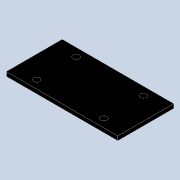
# Autodesk Inventor part: X Axis Belt Tentoner NON ADJUSTABLE Top
Saved by Autodesk Inventor 2022 (Build 260153000, 153)
## iProperties
Created: 2021-10-23
Part Number: X Axis Belt Tentoner NON ADJUSTABLE Top
Material: Generic
Document SubType Name: Modeling
Designer: Coy
Density: 1 g/cm^3
Appearance: Anodized - Black
Author: Coy
Autodesk Inventor part; units mm, degrees
ref_plane "YZ Plane" through (0, 0, 0) normal (1, 0, 0) x (0, 1, 0)
ref_plane "XZ Plane" through (0, 0, 0) normal (0, 1, 0) x (-1, 0, 0)
ref_plane "XY Plane" through (0, 0, 0) normal (0, 0, 1) x (1, 0, 0)
sketch "Sketch1" plane through (0, 0, 0) normal (0, 1, 0) x (-1, 0, 0)
  line L0 (0, 0) -> (93, 0)
  line L1 (93, 0) -> (93, 46.65)
  line L2 (93, 46.65) -> (0, 46.65)
  line L3 (0, 46.65) -> (0, 0)
  line L4 (74.5, 39.825) -> (18.5, 39.825) construction
  line L5 (18.5, 39.825) -> (18.5, 6.825) construction
  line L6 (18.5, 6.825) -> (74.5, 6.825) construction
  line L7 (74.5, 6.825) -> (74.5, 39.825) construction
  line L8 (74.5, 39.825) -> (93, 39.825) construction
  line L9 (74.5, 39.825) -> (74.5, 46.65) construction
  line L10 (18.5, 6.825) -> (18.5, 0) construction
  line L11 (18.5, 6.825) -> (0, 6.825) construction
  circle A0 centre (74.5, 39.825) radius 2.6
  circle A1 centre (74.5, 6.825) radius 2.6
  circle A2 centre (18.5, 6.825) radius 2.6
  circle A3 centre (18.5, 39.825) radius 2.6
  dimension "d0" = 46.65
  dimension "d1" = 93
  dimension "d2" = 33
  dimension "d3" = 56
  dimension "d4" = 5.2
  dimension "d5" = 5.2
  dimension "d6" = 5.2
  dimension "d7" = 5.2
  constraints: 24 end point, 6 parallel, 6 perpendicular, 4 centre point, 4 coincident, 4 point on line, 2 horizontal
  measures "d0" distance of L1.end L0.end
  measures "d1" distance of L1.end L2.end
  measures "d2" distance of L6.end L4.start
  measures "d3" distance of L4.start L4.end
  measures "d4" diameter of A0
  measures "d5" diameter of A1
  measures "d6" diameter of A2
  measures "d7" diameter of A3
extrude "Extrusion1" add sketch "Sketch1" along normal blind 3.5
chamfer "Chamfer1" distance 0.325 angle 45 2 edges at (-93, 1.75, 46.65) (-93, 1.75, 0)
equation "\"d5\" = d4"
equation "\"d6\" = d4"
equation "\"d7\" = d4"
body "Solid1"
